Autodesk Fusion 360 part; units mm, degrees
(part 11 of 11)
  spline S48 degree 5 poles (-71.9508, 42.1491) (-71.9808, 42.1663) (-72.0413, 42.1999) (-72.1332, 42.2481) (-72.2578, 42.3082) (-72.4164, 42.3774) (-72.5771, 42.4424) (-72.7391, 42.5049) (-72.9018, 42.5659) (-73.0649, 42.6261) (-73.2285, 42.6852) (-73.3927, 42.743) (-73.5577, 42.799) (-73.7236, 42.853) (-73.8904, 42.9049) (-74.0581, 42.955) (-74.2265, 43.0033) (-74.3955, 43.0504) (-74.565, 43.0962) (-74.7349, 43.1409) (-74.9053, 43.1845) (-75.0761, 43.2269) (-75.2475, 43.268) (-75.4193, 43.3078) (-75.5917, 43.3463) (-75.7646, 43.3837) (-75.9378, 43.4198) (-76.1116, 43.4548) (-76.2856, 43.4888) (-76.4601, 43.5217) (-76.635, 43.5536) (-76.8102, 43.5844) (-76.9858, 43.6142) (-77.1617, 43.643) (-77.338, 43.6707) (-77.5146, 43.6974) (-77.6916, 43.7231) (-77.8689, 43.7478) (-78.0465, 43.7716) (-78.2244, 43.7945) (-78.4026, 43.8163) (-78.5811, 43.8373) (-78.7599, 43.8573) (-78.939, 43.8764) (-79.1183, 43.8946) (-79.2979, 43.9119) (-79.4778, 43.9283) (-79.658, 43.9438) (-79.8383, 43.9584) (-80.019, 43.9722) (-80.1998, 43.985) (-80.381, 43.9971) (-80.5623, 44.0083) (-80.7439, 44.0186) (-80.9257, 44.0281) (-81.1077, 44.0367) (-81.2899, 44.0445) (-81.4723, 44.0515) (-81.6549, 44.0577) (-81.8378, 44.0631) (-82.0208, 44.0677) (-82.204, 44.0714) (-82.3874, 44.0744) (-82.571, 44.0765) (-82.7548, 44.0779) (-82.9387, 44.0785) (-83.1228, 44.0783) (-83.3071, 44.0773) (-83.4916, 44.0756) (-83.6762, 44.0731) (-83.861, 44.0698) (-84.0089, 44.0665) (-84.1199, 44.0638) (-84.194, 44.0618) (-84.231, 44.0607) knots 0 0 0 0 0 0 0.01428571 0.02857143 0.04285714 0.05714286 0.07142857 0.08571429 0.1 0.11428571 0.12857143 0.14285714 0.15714286 0.17142857 0.18571429 0.2 0.21428571 0.22857143 0.24285714 0.25714286 0.27142857 0.28571429 0.3 0.31428571 0.32857143 0.34285714 0.35714286 0.37142857 0.38571429 0.4 0.41428571 0.42857143 0.44285714 0.45714286 0.47142857 0.48571429 0.5 0.51428571 0.52857143 0.54285714 0.55714286 0.57142857 0.58571429 0.6 0.61428571 0.62857143 0.64285714 0.65714286 0.67142857 0.68571429 0.7 0.71428571 0.72857143 0.74285714 0.75714286 0.77142857 0.78571429 0.8 0.81428571 0.82857143 0.84285714 0.85714286 0.87142857 0.88571429 0.9 0.91428571 0.92857143 0.94285714 0.95714286 0.97142857 0.98571429 1 1 1 1 1 1
  arc A102 (-84.231, 44.0607) -> (-86.2449, 39.8789) centre (0.5538, 0.6546) ccw
  spline S49 degree 5 poles (-77.0937, 31.4697) (-77.1259, 31.4825) (-77.1899, 31.5088) (-77.2849, 31.5505) (-77.4095, 31.6105) (-77.5625, 31.6914) (-77.7135, 31.7765) (-77.8634, 31.8642) (-78.0125, 31.9533) (-78.1613, 32.0433) (-78.3095, 32.1344) (-78.4571, 32.2267) (-78.6037, 32.3207) (-78.7494, 32.4168) (-78.894, 32.5149) (-79.0377, 32.6148) (-79.1805, 32.7163) (-79.3226, 32.8191) (-79.4641, 32.923) (-79.605, 33.028) (-79.7453, 33.134) (-79.885, 33.2412) (-80.024, 33.3495) (-80.1623, 33.4591) (-80.2999, 33.5698) (-80.4368, 33.6817) (-80.5731, 33.7946) (-80.7088, 33.9086) (-80.8439, 34.0235) (-80.9784, 34.1394) (-81.1124, 34.2562) (-81.2457, 34.374) (-81.3785, 34.4927) (-81.5106, 34.6123) (-81.6422, 34.7329) (-81.7732, 34.8543) (-81.9037, 34.9766) (-82.0336, 35.0998) (-82.1629, 35.2239) (-82.2917, 35.3487) (-82.4199, 35.4744) (-82.5476, 35.6009) (-82.6747, 35.7282) (-82.8013, 35.8563) (-82.9273, 35.9852) (-83.0528, 36.1148) (-83.1778, 36.2452) (-83.3022, 36.3764) (-83.4261, 36.5083) (-83.5495, 36.641) (-83.6723, 36.7743) (-83.7947, 36.9084) (-83.9165, 37.0433) (-84.0377, 37.1788) (-84.1585, 37.315) (-84.2787, 37.4519) (-84.3985, 37.5895) (-84.5177, 37.7277) (-84.6364, 37.8667) (-84.7546, 38.0063) (-84.8723, 38.1465) (-84.9894, 38.2874) (-85.1061, 38.429) (-85.2222, 38.5712) (-85.3379, 38.714) (-85.453, 38.8574) (-85.5677, 39.0015) (-85.6818, 39.1462) (-85.7955, 39.2915) (-85.9086, 39.4374) (-86.0212, 39.5839) (-86.111, 39.7016) (-86.178, 39.7901) (-86.2226, 39.8493) (-86.2449, 39.8789) knots 0 0 0 0 0 0 0.01428571 0.02857143 0.04285714 0.05714286 0.07142857 0.08571429 0.1 0.11428571 0.12857143 0.14285714 0.15714286 0.17142857 0.18571429 0.2 0.21428571 0.22857143 0.24285714 0.25714286 0.27142857 0.28571429 0.3 0.31428571 0.32857143 0.34285714 0.35714286 0.37142857 0.38571429 0.4 0.41428571 0.42857143 0.44285714 0.45714286 0.47142857 0.48571429 0.5 0.51428571 0.52857143 0.54285714 0.55714286 0.57142857 0.58571429 0.6 0.61428571 0.62857143 0.64285714 0.65714286 0.67142857 0.68571429 0.7 0.71428571 0.72857143 0.74285714 0.75714286 0.77142857 0.78571429 0.8 0.81428571 0.82857143 0.84285714 0.85714286 0.87142857 0.88571429 0.9 0.91428571 0.92857143 0.94285714 0.95714286 0.97142857 0.98571429 1 1 1 1 1 1
  line L49 (-77.0937, 31.4697) -> (-75.7049, 30.9183)
  arc A103 (-75.2572, 29.8949) -> (-75.7049, 30.9183) centre (-75.9978, 30.1805) ccw
  arc A104 (-75.2572, 29.8949) -> (-76.9486, 25.0611) centre (0.5538, 0.6546) ccw
  arc A105 (-77.9367, 24.5401) -> (-76.9486, 25.0611) centre (-77.7057, 25.2995) ccw
  line L50 (-77.9367, 24.5401) -> (-79.3663, 24.9749)
  spline S50 degree 5 poles (-79.3663, 24.9749) (-79.3995, 24.985) (-79.4659, 25.0043) (-79.5662, 25.0309) (-79.701, 25.0617) (-79.8711, 25.0939) (-80.0422, 25.1215) (-80.214, 25.1464) (-80.3862, 25.1697) (-80.5586, 25.192) (-80.7313, 25.2133) (-80.9042, 25.2331) (-81.0775, 25.251) (-81.2513, 25.2667) (-81.4255, 25.2802) (-81.6002, 25.2917) (-81.7751, 25.3014) (-81.9503, 25.3096) (-82.1257, 25.3166) (-82.3013, 25.3224) (-82.4771, 25.3269) (-82.6531, 25.3302) (-82.8293, 25.3322) (-83.0058, 25.3328) (-83.1824, 25.332) (-83.3592, 25.3299) (-83.5362, 25.3266) (-83.7133, 25.3221) (-83.8906, 25.3165) (-84.068, 25.3097) (-84.2456, 25.3019) (-84.4233, 25.293) (-84.6011, 25.283) (-84.779, 25.2718) (-84.9571, 25.2596) (-85.1352, 25.2464) (-85.3135, 25.232) (-85.4918, 25.2167) (-85.6703, 25.2004) (-85.8488, 25.183) (-86.0274, 25.1647) (-86.2061, 25.1454) (-86.3849, 25.1252) (-86.5637, 25.1039) (-86.7426, 25.0818) (-86.9215, 25.0586) (-87.1006, 25.0346) (-87.2796, 25.0096) (-87.4587, 24.9837) (-87.6379, 24.957) (-87.8171, 24.9293) (-87.9964, 24.9007) (-88.1756, 24.8712) (-88.3549, 24.8409) (-88.5343, 24.8097) (-88.7137, 24.7777) (-88.893, 24.7447) (-89.0725, 24.711) (-89.2519, 24.6763) (-89.4313, 24.6409) (-89.6108, 24.6046) (-89.7902, 24.5675) (-89.9697, 24.5296) (-90.1492, 24.4908) (-90.3286, 24.4513) (-90.5081, 24.4109) (-90.6876, 24.3697) (-90.867, 24.3278) (-91.0464, 24.2851) (-91.2259, 24.2415) (-91.4053, 24.1972) (-91.5488, 24.1611) (-91.6564, 24.1337) (-91.7282, 24.1153) (-91.7641, 24.1061) knots 0 0 0 0 0 0 0.01428571 0.02857143 0.04285714 0.05714286 0.07142857 0.08571429 0.1 0.11428571 0.12857143 0.14285714 0.15714286 0.17142857 0.18571429 0.2 0.21428571 0.22857143 0.24285714 0.25714286 0.27142857 0.28571429 0.3 0.31428571 0.32857143 0.34285714 0.35714286 0.37142857 0.38571429 0.4 0.41428571 0.42857143 0.44285714 0.45714286 0.47142857 0.48571429 0.5 0.51428571 0.52857143 0.54285714 0.55714286 0.57142857 0.58571429 0.6 0.61428571 0.62857143 0.64285714 0.65714286 0.67142857 0.68571429 0.7 0.71428571 0.72857143 0.74285714 0.75714286 0.77142857 0.78571429 0.8 0.81428571 0.82857143 0.84285714 0.85714286 0.87142857 0.88571429 0.9 0.91428571 0.92857143 0.94285714 0.95714286 0.97142857 0.98571429 1 1 1 1 1 1
  arc A106 (-91.7641, 24.1061) -> (-92.7969, 19.5809) centre (0.5538, 0.6546) ccw
  spline S51 degree 5 poles (-82.0039, 13.4189) (-82.0381, 13.4242) (-82.1064, 13.4356) (-82.2083, 13.4551) (-82.3431, 13.4859) (-82.5103, 13.5307) (-82.6765, 13.5801) (-82.8421, 13.6322) (-83.0073, 13.6859) (-83.1724, 13.7406) (-83.3371, 13.7963) (-83.5015, 13.8535) (-83.6655, 13.9126) (-83.8288, 13.9738) (-83.9917, 14.0373) (-84.154, 14.1027) (-84.3158, 14.1699) (-84.4772, 14.2385) (-84.6383, 14.3083) (-84.799, 14.3793) (-84.9594, 14.4515) (-85.1194, 14.5248) (-85.279, 14.5995) (-85.4382, 14.6756) (-85.597, 14.7529) (-85.7554, 14.8315) (-85.9134, 14.9113) (-86.0711, 14.9922) (-86.2284, 15.0742) (-86.3853, 15.1572) (-86.5419, 15.2413) (-86.6981, 15.3264) (-86.8539, 15.4126) (-87.0094, 15.4998) (-87.1645, 15.5881) (-87.3193, 15.6774) (-87.4737, 15.7676) (-87.6277, 15.8588) (-87.7814, 15.9509) (-87.9347, 16.044) (-88.0877, 16.138) (-88.2403, 16.2329) (-88.3926, 16.3287) (-88.5445, 16.4255) (-88.6961, 16.5231) (-88.8473, 16.6215) (-88.9981, 16.7209) (-89.1486, 16.8211) (-89.2988, 16.9221) (-89.4486, 17.024) (-89.598, 17.1267) (-89.7471, 17.2302) (-89.8958, 17.3345) (-90.0442, 17.4396) (-90.1923, 17.5456) (-90.34, 17.6523) (-90.4873, 17.7598) (-90.6343, 17.868) (-90.7809, 17.9771) (-90.9272, 18.0869) (-91.0732, 18.1974) (-91.2188, 18.3087) (-91.364, 18.4208) (-91.5089, 18.5335) (-91.6534, 18.647) (-91.7976, 18.7613) (-91.9414, 18.8762) (-92.0849, 18.9919) (-92.228, 19.1082) (-92.3708, 19.2253) (-92.5132, 19.3431) (-92.6269, 19.4379) (-92.7119, 19.5092) (-92.7686, 19.557) (-92.7969, 19.5809) knots 0 0 0 0 0 0 0.01428571 0.02857143 0.04285714 0.05714286 0.07142857 0.08571429 0.1 0.11428571 0.12857143 0.14285714 0.15714286 0.17142857 0.18571429 0.2 0.21428571 0.22857143 0.24285714 0.25714286 0.27142857 0.28571429 0.3 0.31428571 0.32857143 0.34285714 0.35714286 0.37142857 0.38571429 0.4 0.41428571 0.42857143 0.44285714 0.45714286 0.47142857 0.48571429 0.5 0.51428571 0.52857143 0.54285714 0.55714286 0.57142857 0.58571429 0.6 0.61428571 0.62857143 0.64285714 0.65714286 0.67142857 0.68571429 0.7 0.71428571 0.72857143 0.74285714 0.75714286 0.77142857 0.78571429 0.8 0.81428571 0.82857143 0.84285714 0.85714286 0.87142857 0.88571429 0.9 0.91428571 0.92857143 0.94285714 0.95714286 0.97142857 0.98571429 1 1 1 1 1 1
  line L51 (-82.0039, 13.4189) -> (-80.5272, 13.1903)
  arc A107 (-79.8631, 12.2922) -> (-80.5272, 13.1903) centre (-80.6486, 12.4059) ccw
  arc A108 (-79.8631, 12.2922) -> (-80.4364, 7.2033) centre (0.5538, 0.6546) ccw
  arc A109 (-81.2838, 6.4755) -> (-80.4364, 7.2033) centre (-81.2276, 7.2672) ccw
  line L52 (-81.2838, 6.4755) -> (-82.7743, 6.5813)
  spline S52 degree 5 poles (-82.7743, 6.5813) (-82.8089, 6.5837) (-82.878, 6.5878) (-82.9816, 6.5914) (-83.1199, 6.5914) (-83.2929, 6.5849) (-83.4659, 6.5738) (-83.6389, 6.5598) (-83.812, 6.5442) (-83.9851, 6.5276) (-84.1581, 6.5099) (-84.3311, 6.4908) (-84.5041, 6.4697) (-84.677, 6.4463) (-84.8498, 6.4207) (-85.0226, 6.393) (-85.1954, 6.3635) (-85.368, 6.3326) (-85.5406, 6.3003) (-85.7131, 6.2669) (-85.8855, 6.2322) (-86.0578, 6.1963) (-86.23, 6.159) (-86.4021, 6.1203) (-86.5742, 6.0802) (-86.7461, 6.0388) (-86.9179, 5.9962) (-87.0896, 5.9524) (-87.2612, 5.9075) (-87.4327, 5.8615) (-87.604, 5.8143) (-87.7753, 5.7661) (-87.9464, 5.7167) (-88.1174, 5.6663) (-88.2882, 5.6148) (-88.459, 5.5622) (-88.6296, 5.5086) (-88.8001, 5.4539) (-88.9704, 5.3983) (-89.1406, 5.3417) (-89.3106, 5.2841) (-89.4806, 5.2255) (-89.6503, 5.166) (-89.8199, 5.1055) (-89.9894, 5.044) (-90.1588, 4.9817) (-90.3279, 4.9184) (-90.4969, 4.8542) (-90.6658, 4.7891) (-90.8345, 4.7231) (-91.0031, 4.6563) (-91.1715, 4.5885) (-91.3397, 4.5199) (-91.5078, 4.4504) (-91.6757, 4.3801) (-91.8434, 4.3089) (-92.011, 4.2369) (-92.1784, 4.1641) (-92.3456, 4.0904) (-92.5127, 4.0159) (-92.6795, 3.9406) (-92.8462, 3.8645) (-93.0128, 3.7876) (-93.1791, 3.7099) (-93.3453, 3.6314) (-93.5113, 3.5521) (-93.6771, 3.472) (-93.8427, 3.3912) (-94.0081, 3.3096) (-94.1733, 3.2272) (-94.3384, 3.1441) (-94.4703, 3.077) (-94.5691, 3.0263) (-94.635, 2.9924) (-94.6679, 2.9754) knots 0 0 0 0 0 0 0.01428571 0.02857143 0.04285714 0.05714286 0.07142857 0.08571429 0.1 0.11428571 0.12857143 0.14285714 0.15714286 0.17142857 0.18571429 0.2 0.21428571 0.22857143 0.24285714 0.25714286 0.27142857 0.28571429 0.3 0.31428571 0.32857143 0.34285714 0.35714286 0.37142857 0.38571429 0.4 0.41428571 0.42857143 0.44285714 0.45714286 0.47142857 0.48571429 0.5 0.51428571 0.52857143 0.54285714 0.55714286 0.57142857 0.58571429 0.6 0.61428571 0.62857143 0.64285714 0.65714286 0.67142857 0.68571429 0.7 0.71428571 0.72857143 0.74285714 0.75714286 0.77142857 0.78571429 0.8 0.81428571 0.82857143 0.84285714 0.85714286 0.87142857 0.88571429 0.9 0.91428571 0.92857143 0.94285714 0.95714286 0.97142857 0.98571429 1 1 1 1 1 1
  arc A110 (-94.6679, 2.9754) -> (-94.6679, -1.6661) centre (0.5538, 0.6546) ccw
  spline S53 degree 5 poles (-82.7743, -5.272) (-82.8089, -5.2744) (-82.878, -5.2785) (-82.9816, -5.2821) (-83.1199, -5.2821) (-83.2929, -5.2756) (-83.4659, -5.2645) (-83.6389, -5.2505) (-83.812, -5.2349) (-83.9851, -5.2183) (-84.1581, -5.2006) (-84.3311, -5.1815) (-84.5041, -5.1604) (-84.677, -5.137) (-84.8498, -5.1114) (-85.0226, -5.0837) (-85.1954, -5.0542) (-85.368, -5.0233) (-85.5406, -4.991) (-85.7131, -4.9576) (-85.8855, -4.9229) (-86.0578, -4.887) (-86.23, -4.8497) (-86.4021, -4.811) (-86.5742, -4.7709) (-86.7461, -4.7296) (-86.9179, -4.6869) (-87.0896, -4.6431) (-87.2612, -4.5982) (-87.4327, -4.5522) (-87.604, -4.505) (-87.7753, -4.4568) (-87.9464, -4.4075) (-88.1174, -4.357) (-88.2882, -4.3055) (-88.459, -4.2529) (-88.6296, -4.1993) (-88.8001, -4.1446) (-88.9704, -4.089) (-89.1406, -4.0324) (-89.3106, -3.9748) (-89.4806, -3.9162) (-89.6503, -3.8567) (-89.8199, -3.7962) (-89.9894, -3.7348) (-90.1588, -3.6724) (-90.3279, -3.6091) (-90.4969, -3.5449) (-90.6658, -3.4798) (-90.8345, -3.4139) (-91.0031, -3.347) (-91.1715, -3.2793) (-91.3397, -3.2106) (-91.5078, -3.1412) (-91.6757, -3.0708) (-91.8434, -2.9997) (-92.011, -2.9277) (-92.1784, -2.8548) (-92.3456, -2.7811) (-92.5127, -2.7067) (-92.6795, -2.6313) (-92.8462, -2.5552) (-93.0128, -2.4783) (-93.1791, -2.4006) (-93.3453, -2.3221) (-93.5113, -2.2428) (-93.6771, -2.1628) (-93.8427, -2.0819) (-94.0081, -2.0003) (-94.1733, -1.918) (-94.3384, -1.8348) (-94.4703, -1.7677) (-94.5691, -1.7171) (-94.635, -1.6831) (-94.6679, -1.6661) knots 0 0 0 0 0 0 0.01428571 0.02857143 0.04285714 0.05714286 0.07142857 0.08571429 0.1 0.11428571 0.12857143 0.14285714 0.15714286 0.17142857 0.18571429 0.2 0.21428571 0.22857143 0.24285714 0.25714286 0.27142857 0.28571429 0.3 0.31428571 0.32857143 0.34285714 0.35714286 0.37142857 0.38571429 0.4 0.41428571 0.42857143 0.44285714 0.45714286 0.47142857 0.48571429 0.5 0.51428571 0.52857143 0.54285714 0.55714286 0.57142857 0.58571429 0.6 0.61428571 0.62857143 0.64285714 0.65714286 0.67142857 0.68571429 0.7 0.71428571 0.72857143 0.74285714 0.75714286 0.77142857 0.78571429 0.8 0.81428571 0.82857143 0.84285714 0.85714286 0.87142857 0.88571429 0.9 0.91428571 0.92857143 0.94285714 0.95714286 0.97142857 0.98571429 1 1 1 1 1 1
  line L53 (-82.7743, -5.272) -> (-81.2838, -5.1662)
  arc A111 (-80.4364, -5.894) -> (-81.2838, -5.1662) centre (-81.2276, -5.958) ccw
  arc A112 (-80.4364, -5.894) -> (-79.8631, -10.983) centre (0.5538, 0.6546) ccw
  arc A113 (-80.5272, -11.8811) -> (-79.8631, -10.983) centre (-80.6486, -11.0966) ccw
  line L54 (-80.5272, -11.8811) -> (-82.0039, -12.1096)
  spline S54 degree 5 poles (-82.0039, -12.1096) (-82.0381, -12.1149) (-82.1064, -12.1263) (-82.2083, -12.1459) (-82.3431, -12.1766) (-82.5103, -12.2214) (-82.6765, -12.2708) (-82.8421, -12.3229) (-83.0073, -12.3766) (-83.1724, -12.4313) (-83.3371, -12.4871) (-83.5015, -12.5442) (-83.6655, -12.6033) (-83.8288, -12.6646) (-83.9917, -12.728) (-84.154, -12.7934) (-84.3158, -12.8606) (-84.4772, -12.9292) (-84.6383, -12.999) (-84.799, -13.07) (-84.9594, -13.1422) (-85.1194, -13.2156) (-85.279, -13.2903) (-85.4382, -13.3663) (-85.597, -13.4436) (-85.7554, -13.5222) (-85.9134, -13.602) (-86.0711, -13.6829) (-86.2284, -13.7649) (-86.3853, -13.8479) (-86.5419, -13.932) (-86.6981, -14.0172) (-86.8539, -14.1033) (-87.0094, -14.1906) (-87.1645, -14.2788) (-87.3193, -14.3681) (-87.4737, -14.4583) (-87.6277, -14.5495) (-87.7814, -14.6417) (-87.9347, -14.7347) (-88.0877, -14.8287) (-88.2403, -14.9236) (-88.3926, -15.0195) (-88.5445, -15.1162) (-88.6961, -15.2138) (-88.8473, -15.3123) (-88.9981, -15.4116) (-89.1486, -15.5118) (-89.2988, -15.6128) (-89.4486, -15.7147) (-89.598, -15.8174) (-89.7471, -15.9209) (-89.8958, -16.0252) (-90.0442, -16.1304) (-90.1923, -16.2363) (-90.34, -16.343) (-90.4873, -16.4505) (-90.6343, -16.5588) (-90.7809, -16.6678) (-90.9272, -16.7776) (-91.0732, -16.8881) (-91.2188, -16.9994) (-91.364, -17.1115) (-91.5089, -17.2243) (-91.6534, -17.3378) (-91.7976, -17.452) (-91.9414, -17.5669) (-92.0849, -17.6826) (-92.228, -17.799) (-92.3708, -17.916) (-92.5132, -18.0338) (-92.6269, -18.1286) (-92.7119, -18.2) (-92.7686, -18.2477) (-92.7969, -18.2716) knots 0 0 0 0 0 0 0.01428571 0.02857143 0.04285714 0.05714286 0.07142857 0.08571429 0.1 0.11428571 0.12857143 0.14285714 0.15714286 0.17142857 0.18571429 0.2 0.21428571 0.22857143 0.24285714 0.25714286 0.27142857 0.28571429 0.3 0.31428571 0.32857143 0.34285714 0.35714286 0.37142857 0.38571429 0.4 0.41428571 0.42857143 0.44285714 0.45714286 0.47142857 0.48571429 0.5 0.51428571 0.52857143 0.54285714 0.55714286 0.57142857 0.58571429 0.6 0.61428571 0.62857143 0.64285714 0.65714286 0.67142857 0.68571429 0.7 0.71428571 0.72857143 0.74285714 0.75714286 0.77142857 0.78571429 0.8 0.81428571 0.82857143 0.84285714 0.85714286 0.87142857 0.88571429 0.9 0.91428571 0.92857143 0.94285714 0.95714286 0.97142857 0.98571429 1 1 1 1 1 1
  arc A114 (-92.7969, -18.2716) -> (-91.7641, -22.7968) centre (0.5538, 0.6546) ccw
  spline S55 degree 5 poles (-79.3663, -23.6657) (-79.3995, -23.6757) (-79.4659, -23.6951) (-79.5662, -23.7216) (-79.701, -23.7524) (-79.8711, -23.7846) (-80.0422, -23.8122) (-80.214, -23.8371) (-80.3862, -23.8604) (-80.5586, -23.8828) (-80.7313, -23.904) (-80.9042, -23.9238) (-81.0775, -23.9417) (-81.2513, -23.9575) (-81.4255, -23.9709) (-81.6002, -23.9824) (-81.7751, -23.9921) (-81.9503, -24.0003) (-82.1257, -24.0073) (-82.3013, -24.0131) (-82.4771, -24.0177) (-82.6531, -24.021) (-82.8293, -24.0229) (-83.0058, -24.0235) (-83.1824, -24.0227) (-83.3592, -24.0206) (-83.5362, -24.0173) (-83.7133, -24.0128) (-83.8906, -24.0072) (-84.068, -24.0005) (-84.2456, -23.9926) (-84.4233, -23.9837) (-84.6011, -23.9737) (-84.779, -23.9626) (-84.9571, -23.9504) (-85.1352, -23.9371) (-85.3135, -23.9228) (-85.4918, -23.9074) (-85.6703, -23.8911) (-85.8488, -23.8738) (-86.0274, -23.8554) (-86.2061, -23.8361) (-86.3849, -23.8159) (-86.5637, -23.7947) (-86.7426, -23.7725) (-86.9215, -23.7494) (-87.1006, -23.7253) (-87.2796, -23.7003) (-87.4587, -23.6745) (-87.6379, -23.6477) (-87.8171, -23.62) (-87.9964, -23.5914) (-88.1756, -23.562) (-88.3549, -23.5316) (-88.5343, -23.5004) (-88.7137, -23.4684) (-88.893, -23.4355) (-89.0725, -23.4017) (-89.2519, -23.3671) (-89.4313, -23.3316) (-89.6108, -23.2953) (-89.7902, -23.2582) (-89.9697, -23.2203) (-90.1492, -23.1815) (-90.3286, -23.142) (-90.5081, -23.1016) (-90.6876, -23.0605) (-90.867, -23.0185) (-91.0464, -22.9758) (-91.2259, -22.9322) (-91.4053, -22.8879) (-91.5488, -22.8519) (-91.6564, -22.8245) (-91.7282, -22.806) (-91.7641, -22.7968) knots 0 0 0 0 0 0 0.01428571 0.02857143 0.04285714 0.05714286 0.07142857 0.08571429 0.1 0.11428571 0.12857143 0.14285714 0.15714286 0.17142857 0.18571429 0.2 0.21428571 0.22857143 0.24285714 0.25714286 0.27142857 0.28571429 0.3 0.31428571 0.32857143 0.34285714 0.35714286 0.37142857 0.38571429 0.4 0.41428571 0.42857143 0.44285714 0.45714286 0.47142857 0.48571429 0.5 0.51428571 0.52857143 0.54285714 0.55714286 0.57142857 0.58571429 0.6 0.61428571 0.62857143 0.64285714 0.65714286 0.67142857 0.68571429 0.7 0.71428571 0.72857143 0.74285714 0.75714286 0.77142857 0.78571429 0.8 0.81428571 0.82857143 0.84285714 0.85714286 0.87142857 0.88571429 0.9 0.91428571 0.92857143 0.94285714 0.95714286 0.97142857 0.98571429 1 1 1 1 1 1
  line L55 (-79.3663, -23.6657) -> (-77.9367, -23.2308)
  arc A115 (-76.9486, -23.7518) -> (-77.9367, -23.2308) centre (-77.7057, -23.9902) ccw
  arc A116 (-76.9486, -23.7518) -> (-75.2572, -28.5856) centre (0.5538, 0.6546) ccw
  circle A117 centre (0.5538, 0.6546) radius 95.3499
  dimension "d117" = 79.8499
extrude "Extrude5" add sketch "Sketch5" along normal blind 10 contours A5 L0 S0 A6 S1 L1 A7 A8 A9 L2 S2 A10 S3 L3 A11 A12 A13 L4 S4 A14 S5 L5 A15 A16 A17 L6 S6 A18 S7 L7 A19 A20 A21 L8 S8 A22 S9 L9 A23 A24 A25 L10 S10 A26 S11 L11 A27 A28 A29 L12 S12 A30 S13 L13 A31 A32 A33 L14 S14 A34 S15 L15 A35 A36 A37 L16 S16 A38 S17 L17 A39 A40 A41 L18 S18 A42 S19 L19 A43 A44 A45 L20 S20 A46 S21 L21 A47 A48 A49 L22 S22 A50 S23 L23 A51 A52 A53 L24 S24 A54 S25 L25 A55 A56 A57 L26 S26 A58 S27 L27 A59 A60 A61 L28 S28 A62 S29 L29 A63 A64 A65 L30 S30 A66 S31 L31 A67 A68 A69 L32 S32 A70 S33 L33 A71 A72 A73 L34 S34 A74 S35 L35 A75 A76 A77 L36 S36 A78 S37 L37 A79 A80 A81 L38 S38 A82 S39 L39 A83 A84 A85 L40 S40 A86 S41 L41 A87 A88 A89 L42 S42 A90 S43 L43 A91 A92 A93 L44 S44 A94 S45 L45 A95 A96 A97 L46 S46 A98 S47 L47 A99 A100 A101 L48 S48 A102 S49 L49 A103 A104 A105 L50 S50 A106 S51 L51 A107 A108 A109 L52 S52 A110 S53 L53 A111 A112 A113 L54 S54 A114 S55 L55 A115 A116 | A117 sketch seen with x (1, 0, 0) y (0, 1, 0) z (0, 0, 1) at (-80.4364, -7.2033, 0) bodies 1 in component "Spur Gear (28 teeth)"
extrude "Extrude6" cut 1 faces at (-46.0448, 29.3999, 2.5) along direction (0, 0, 1) blind 5 on bodies 1 bodies 1 in component "Spur Gear (28 teeth)"
sketch "Sketch6" plane through (0, -107.79, 0) normal (0, -1, 0) x (1, 0, 0)
  line L0 (-102.9957, 25) -> (-82.9957, 25)
  line L1 (-82.9957, 25) -> (-82.9957, 45)
  line L2 (-82.9957, 45) -> (-102.9957, 45)
  line L3 (-102.9957, 45) -> (-102.9957, 25)
  line L4 (-102.9957, 45) -> (-82.9957, 25) construction
  line L5 (-82.9957, 45) -> (-102.9957, 25) construction
  circle A0 centre (-92.9957, 35) radius 2.25
  dimension "d122" = 4.5
  constraint coincident L2.end L3.start
  constraint coincident L0.end L1.start
  constraint coincident L1.end L2.start
  constraint coincident L0.start L3.end
  constraint midpoint L5 A0.centre
  measures "d122" diameter of A0
extrude "Extrude4'" cut sketch "Sketch6" against normal blind 34 contours A0 sketch seen with x (1, 0, 0) y (0, 1, 0) z (0, 0, 1) at (12.0054, 91.2413, 0) bodies 2 in component "Spur Gear (14 teeth)"
sketch "Sketch7" plane through (0, 0, 45) normal (0, 0, 1) x (1, 0, 0)
  circle A0 centre (-92.9957, -97.79) radius 5
  line L0 (-102.9957, -107.79) -> (-82.9957, -107.79)
  line L1 (-82.9957, -107.79) -> (-82.9957, -87.79)
  line L2 (-82.9957, -87.79) -> (-102.9957, -87.79)
  line L3 (-102.9957, -87.79) -> (-102.9957, -107.79)
  circle A1 centre (-92.9957, -97.79) radius 2.5
  dimension "d125" = -2.5
extrude "Extrude5'" add sketch "Sketch7" against normal blind 32.5 contours A0 sketch seen with x (1, 0, 0) y (0, 1, 0) z (0, 0, 1) at (12.0054, 91.2413, 0) bodies 2 in component "Spur Gear (14 teeth)"
sketch "Sketch8" plane through (0, 0, 25) normal (0, 0, 1) x (1, 0, 0)
  circle A0 centre (0, 0) radius 70
  circle A1 centre (50, -10) radius 2.75
  circle A2 centre (-50, 10) radius 2.75
  circle A3 centre (50, 10) radius 2.75
  circle A4 centre (-50, -10) radius 2.75
  circle A5 centre (-0.5538, 0.6546) radius 15.5
  circle A6 centre (-0.5538, 0.6546) radius 18.375
  dimension "d128" = 2.875
extrude "Extrude7" cut sketch "Sketch8" against normal blind 40 contours A6 sketch seen with x (1, 0, 0) y (0, 1, 0) z (0, 0, 1) at (-80.4364, -7.2033, 0) bodies 1 in component "Spur Gear (28 teeth)"
extrude "Extrude6'" cut sketch "Sketch6" against normal blind 30 contours A0 sketch seen with x (1, 0, 0) y (0, 1, 0) z (0, 0, 1) at (12.0054, 91.2413, 0) bodies 2 in component "Spur Gear (14 teeth)"
fillet "Fillet2" radius 5 4 edges at (-90.9903, -16.5486, 35) (-70.9903, -16.5486, 35) (-70.9903, 3.4514, 35) (-90.9903, 3.4514, 35) on bodies 2 in component "Spur Gear (14 teeth)"
component "Spur Gear (28 teeth)" placed x (1, 0, 0) y (0, 1, 0) z (0, 0, 1) at (80.4364, 7.2033, 0)
component "Spur Gear (14 teeth)" placed x (1, 0, 0) y (0, 1, 0) z (0, 0, 1) at (-12.0054, -91.2413, 0)
